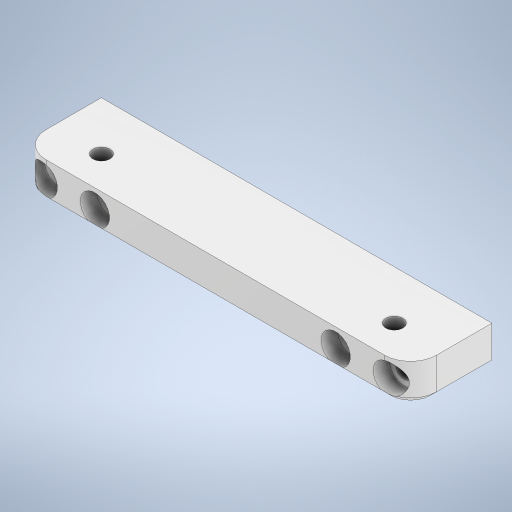
# Autodesk Inventor part: Door Bar Brace Mount
Saved by Autodesk Inventor 2024 (Build 280153000, 153)
## iProperties
Created: 2024-11-21
Part Number: Door Bar Brace Mount
Material: ABS Plastic
Document SubType Name: Modeling
Designer: Ishaan
Density: 1.06 g/cm^3
Appearance: Smooth - White
Author: Ishaan
Autodesk Inventor part; units mm, degrees
ref_plane "YZ Plane" through (0, 0, 0) normal (1, 0, 0) x (0, 1, 0)
ref_plane "XZ Plane" through (0, 0, 0) normal (0, 1, 0) x (-1, 0, 0)
ref_plane "XY Plane" through (0, 0, 0) normal (0, 0, 1) x (1, 0, 0)
sketch "Sketch1" plane through (0, 0, 0) normal (0, 0, 1) x (1, 0, 0)
  line L0 (60, -5.875) -> (-60, -5.875)
  line L1 (-60, -5.875) -> (-60, 5.875)
  line L2 (-60, 5.875) -> (60, 5.875)
  line L3 (60, 5.875) -> (60, -5.875)
  line L4 (60, -5.875) -> (-60, 5.875) construction
  line L5 (-60, -5.875) -> (60, 5.875) construction
  point P0 (0, 0)
  dimension "d0" = 120
  dimension "d1" = 11.75
  constraints: 12 end point, 2 midpoint, 2 parallel, 1 horizontal, 1 perpendicular
  measures "d0" distance of L1.end L2.end
  measures "d1" distance of L0.end L1.end
extrude "Extrusion1" add sketch "Sketch1" along normal blind 25
fillet "Fillet1" radius 8 2 edges at (60, 0, 25) (-60, 0, 25)
chamfer "Chamfer1" distance 2 angle 45 5 edges at (60, -5.875, 8.5) (57.6569, -5.875, 22.6569) (0, -5.875, 25) (-57.6569, -5.875, 22.6569) (-60, -5.875, 8.5)
sketch "Sketch2" plane through (0, 0, 25) normal (0, 0, 1) x (1, 0, 0)
  line L0 (-53, 0.125) -> (-37, 0.125) construction
  line L1 (-52, -5.875) -> (52, -5.875) projected
  line L2 (-60, 5.875) -> (-60, -3.875) projected
  line L3 (37, 0.125) -> (53, 0.125) construction
  line L4 (60, -3.875) -> (60, 5.875) projected
  point P0 (-45, 0.125)
  point P1 (45, 0.125)
  dimension "d8" = 16
  dimension "d9" = 6
  dimension "d35" = 15
  dimension "d36" = 15
  dimension "d37" = 90
  constraints: 4 coincident, 4 end point, 2 collinear, 2 horizontal, 2 midpoint
  measures "d8" distance of L0.start L0.end
  measures "d9" distance between parallel lines of L0 L1
  measures "d35" distance from line of point (-45, 0.125) L2
  measures "d36" distance from line of L4 point (45, 0.125)
  measures "d37" distance of point (-45, 0.125) point (45, 0.125)
hole "Hole1" at (-53, 0.125, 25) at (-37, 0.125, 25) at (37, 0.125, 25) at (53, 0.125, 25) direction (0, 0, -1) diameter 5.3 end through all counterbore diameter 9 counterbore depth 5
sketch "Sketch3" plane through (-60, 5.875, 0) normal (0, 1, 0) x (1, 0, 0)
  point P0 (60, 0)
  point P1 (105, -15)
  point P2 (15, -15)
  point P3 (15, -25)
  point P4 (105, -25)
  dimension "d22" = 10
  constraints: 2 vertical alignment, 1 horizontal alignment
  measures "d22" distance of point (105, -25) point (105, -15)
hole "Hole2" at (45, 5.875, 15) at (-45, 5.875, 15) direction (0, -1, 0) diameter 5.3 end through all
sketch "Sketch4" plane through (-58, -5.875, 0) normal (0, -1, 0) x (1, 0, 0)
  circle A0 centre (13, 15) radius 2.65 projected
  circle A1 centre (103, 15) radius 2.65 projected
  line L0 (0, 0) -> (0, 17) projected
  line L1 (0, 0) -> (116, 0) projected
  line L2 (116, 17) -> (116, 0) projected
  arc A2 (116, 17) -> (110, 23) centre (110, 17) ccw projected
  line L3 (6, 23) -> (110, 23) projected
  arc A3 (6, 23) -> (0, 17) centre (6, 17) ccw projected
  line L4 (107.125, 12.6184) -> (103, 10.2369)
  line L5 (103, 10.2369) -> (98.875, 12.6184)
  line L6 (98.875, 12.6184) -> (98.875, 17.3816)
  line L7 (98.875, 17.3816) -> (103, 19.7631)
  line L8 (103, 19.7631) -> (107.125, 17.3816)
  line L9 (107.125, 17.3816) -> (107.125, 12.6184)
  line L10 (8.875, 17.3816) -> (13, 19.7631)
  line L11 (13, 19.7631) -> (17.125, 17.3816)
  line L12 (17.125, 17.3816) -> (17.125, 12.6184)
  line L13 (17.125, 12.6184) -> (13, 10.2369)
  line L14 (13, 10.2369) -> (8.875, 12.6184)
  line L15 (8.875, 12.6184) -> (8.875, 17.3816)
  point P0 (58, 0)
  dimension "d30" = 8.25
  constraints: 24 end point, 2 coincident, 2 vertical, 1 parallel, 26 other
  measures "d30" distance between parallel lines of L5 L8
extrude "Extrusion2" cut sketch "Sketch4" against normal blind 5 contours A0 | A1 | L4 L5 L6 L7 L8 L9 | L10 L11 L12 L13 L14 L15
equation "\"d35\" = d36"
body "Solid1"
